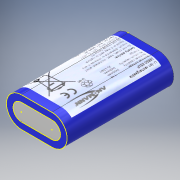
# Autodesk Inventor part: Battery Pack
Saved by Autodesk Inventor 2019 (Build 230136000, 136)
## iProperties
Created: 2020-01-24
Part Number: Battery Pack
Material: Generic
Document SubType Name: Modeling
Designer: pwb15140
Density: 1 g/cm^3
Appearance: Default
Author: pwb15140
Autodesk Inventor part; units mm, degrees
ref_plane "YZ Plane" through (0, 0, 0) normal (1, 0, 0) x (0, 1, 0)
ref_plane "XZ Plane" through (0, 0, 0) normal (0, 1, 0) x (-1, 0, 0)
ref_plane "XY Plane" through (0, 0, 0) normal (0, 0, 1) x (1, 0, 0)
sketch "Sketch1" plane through (0, 0, 0) normal (0, 0, 1) x (1, 0, 0)
  arc A0 (0, 9.2) -> (0, -9.2) centre (0, 0) ccw
  arc A1 (18.6, -9.2) -> (18.6, 9.2) centre (18.6, 0) ccw
  line L0 (0, 9.2) -> (18.6, 9.2)
  line L1 (0, -9.2) -> (18.6, -9.2)
  dimension "d0" = 18.4
  dimension "d1" = 18.4
  dimension "d2" = 18.6
  constraints: 4 end point, 4 point on circle, 2 centre point, 2 tangent, 1 coincident, 1 parallel
  measures "d0" diameter of A0
  measures "d1" diameter of A1
  measures "d2" distance of A1.centre point (0, 0)
extrude "Extrusion1" add sketch "Sketch1" along normal blind 65
sketch "Sketch2" plane through (0, 0, 65) normal (0, 0, 1) x (1, 0, 0)
  line L0 (18.6, 9.2) -> (0, 9.2) projected
  arc A0 (0, 9.2) -> (0, -9.2) centre (0, 0) ccw projected
  line L1 (0, -9.2) -> (18.6, -9.2) projected
  arc A1 (18.6, -9.2) -> (18.6, 9.2) centre (18.6, 0) ccw projected
  line L2 (0, 5.2) -> (18.6, 5.2)
  arc A2 (18.6, -5.2) -> (18.6, 5.2) centre (18.6, 0) ccw
  line L3 (18.6, -5.2) -> (0, -5.2)
  arc A3 (0, 5.2) -> (0, -5.2) centre (0, 0) ccw
  dimension "d7" = 4
  constraints: 4 end point, 4 point on circle, 2 centre point, 3 other
  measures "d7" distance between parallel lines of L0 L2
extrude "Extrusion2" add sketch "Sketch2" along normal blind 0.1
sketch "Sketch3" plane through (0, 0, 0) normal (0, 0, -1) x (-1, 0, 0)
  line L0 (-18.6, 9.2) -> (0, 9.2) projected
  arc A0 (-18.6, 9.2) -> (-18.6, -9.2) centre (-18.6, 0) ccw projected
  line L1 (0, -9.2) -> (-18.6, -9.2) projected
  arc A1 (0, -9.2) -> (0, 9.2) centre (0, 0) ccw projected
  line L2 (0, 5.2) -> (-18.6, 5.2)
  arc A2 (-18.6, 5.2) -> (-18.6, -5.2) centre (-18.6, 0) ccw
  line L3 (-18.6, -5.2) -> (0, -5.2)
  arc A3 (0, -5.2) -> (0, 5.2) centre (0, 0) ccw
  dimension "d8" = 4
  constraints: 4 end point, 4 point on circle, 2 centre point, 3 other
  measures "d8" distance between parallel lines of L0 L2
extrude "Extrusion3" add sketch "Sketch3" along normal blind 0.1
sketch "Sketch4" plane through (0, 9.2, 65.1) normal (0, 1, 0) x (1, 0, 0)
  point P0 (0, 65.1)
sketch "Sketch5" plane through (0, 9.2, 65.1) normal (0, 1, 0) x (1, 0, 0)
  line L0 (25.672, 60.4824) -> (25.672, 5.7019) construction
  line L1 (25.672, 5.7019) -> (-6.5778, 5.7019) construction
  line L2 (-6.5778, 5.7019) -> (-6.5778, 60.4824) construction
  line L3 (-6.5778, 60.4824) -> (25.672, 60.4824) construction
  point P0 (0, 65.1)
  constraints: 2 other
decal "Decal1"
sketch "Sketch6" plane through (0, 0, 65.1) normal (0, 0, 1) x (1, 0, 0)
  arc A0 (18.6, -5.2) -> (18.6, 5.2) centre (18.6, 0) ccw projected
  line L0 (18.6, -5.2) -> (0, -5.2) projected
  arc A1 (0, 5.2) -> (0, -5.2) centre (0, 0) ccw projected
  line L1 (0, 5.2) -> (18.6, 5.2) projected
  line L2 (18.6, 9.2) -> (0, 9.2) projected
  arc A2 (0, 9.2) -> (0, -9.2) centre (0, 0) ccw projected
  line L3 (0, -9.2) -> (18.6, -9.2) projected
  arc A3 (18.6, -9.2) -> (18.6, 9.2) centre (18.6, 0) ccw projected
body "Solid1"
